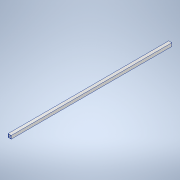
# Autodesk Inventor part: aluprofile_1m
Saved by Autodesk Inventor 2020 (Build 240168000, 168)
## iProperties
Created: 2017-12-03
Part Number: aluprofile_1m
Material: Aluminum 6061
Document SubType Name: Modeling
Designer: stedrock
Density: 2.7 g/cm^3
Appearance: Aluminum - Flat
Mass: 512.325 g
Surface Area: 1383.8 cm^2
Volume: 189.75 cm^3
Author: stedrock
Autodesk Inventor part; units mm, degrees
ref_plane "YZ Plane" through (0, 0, 0) normal (1, 0, 0) x (0, 1, 0)
ref_plane "XZ Plane" through (0, 0, 0) normal (0, 1, 0) x (-1, 0, 0)
ref_plane "XY Plane" through (0, 0, 0) normal (0, 0, 1) x (1, 0, 0)
sketch "Sketch1" plane through (0, 0, 0) normal (0, 0, 1) x (1, 0, 0)
  line L0 (-10, -10) -> (10, -10)
  line L1 (10, -10) -> (10, 10)
  line L2 (10, 10) -> (-10, 10)
  line L3 (-10, 10) -> (-10, -10)
  line L4 (-10, -10) -> (10, 10) construction
  line L5 (10, -10) -> (-10, 10) construction
  line L6 (-7.25, -7.25) -> (7.25, -7.25)
  line L7 (7.25, -7.25) -> (7.25, 7.25)
  line L8 (7.25, 7.25) -> (-7.25, 7.25)
  line L9 (-7.25, 7.25) -> (-7.25, -7.25)
  line L10 (-7.25, -7.25) -> (7.25, 7.25) construction
  line L11 (7.25, -7.25) -> (-7.25, 7.25) construction
  point P0 (0, 0)
  dimension "d0" = 20
  dimension "d1" = 20
  dimension "d2" = 14.5
  dimension "d3" = 14.5
  constraints: 24 end point, 4 equal length, 4 midpoint, 2 perpendicular, 1 horizontal, 1 vertical
  measures "d0" distance of L2.end L1.end
  measures "d1" distance of L1.end L0.end
  measures "d2" distance of L8.end L7.end
  measures "d3" distance of L7.end L6.end
extrude "Extrusion1" add sketch "Sketch1" along normal blind 1000
equation "\"d3\" = d2"
body "Solid1"
